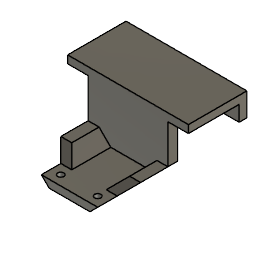
bumper_mount (Autodesk Fusion 360 design; units mm, degrees)
Autodesk Fusion 360 part; units mm, degrees
note: some values were not read from the file. Chosen so that the rebuilt part matches the saved one: which face or edge a step refers to; which pieces of a blend or face edit are solid.
sketch "Sketch1" plane through (0, 0, 0) normal (0, 0, 1) x (1, 0, 0)
  line L0 (-50, 46.2078) -> (-41.5, 46.2078)
  line L1 (-41.5, 46.2078) -> (-41.5, 16.2078)
  line L2 (-41.5, 16.2078) -> (-50, 16.2078)
  line L3 (-50, 16.2078) -> (-50, 46.2078)
  line L4 (-41.5, 16.2078) -> (-0.5, 16.2078)
  line L5 (-0.5, 16.2078) -> (-0.5, 21.2078)
  line L6 (-0.5, 21.2078) -> (-41.5, 21.2078)
  line L7 (-41.5, 21.2078) -> (-41.5, 16.2078)
  line L8 (-0.5, 16.2078) -> (8, 16.2078)
  line L9 (8, 16.2078) -> (8, 46.2078)
  line L10 (8, 46.2078) -> (-0.5, 46.2078)
  line L11 (-0.5, 46.2078) -> (-0.5, 16.2078)
  line L12 (-50, 46.2078) -> (-50, 42.2078)
  line L13 (-50, 42.2078) -> (-41.5, 42.2078)
  line L14 (-0.5, 46.2078) -> (-0.5, 42.2078)
  line L15 (-0.5, 42.2078) -> (8, 42.2078)
  dimension "d1" = 8.5
  dimension "d2" = 30
  dimension "d3" = 41
  dimension "d4" = 5
  dimension "d5" = 8.5
  dimension "d6" = 30
  dimension "d7" = 4
  dimension "d8" = 4
  constraint horizontal L0
  constraint vertical L1
  constraint horizontal L2
  constraint vertical L3
  constraint horizontal L4
  constraint vertical L5
  constraint horizontal L6
  constraint vertical L7
  constraint horizontal L8
  constraint vertical L9
  constraint horizontal L10
  constraint vertical L11
  constraint perpendicular L0 L12
  constraint coincident L1 L13.end
  constraint perpendicular L1 L13
  constraint coincident L11 L14.end
  constraint coincident L9 L15.end
  constraint perpendicular L9 L15
  measures "d1" distance of L0.start L0.end
  measures "d2" distance of L0.start L2.end
  measures "d3" distance of L1.end L4.end
  measures "d4" distance of L1.end L6.end
  measures "d5" distance of L4.end L8.end
  measures "d6" distance of L4.end L10.end
  measures "d7" distance of L0.start L12.end
  measures "d8" distance of L10.end L14.end
extrude "Extrude1" add sketch "Sketch1" against normal blind 8 contours L0 L1 L3 L12 L13 | L9 L10 L11 L14 L15 makes body 1 at (-47.1667, 46.2078, -2.6667) makes body 2 at (5.1667, 46.2078, -2.6667)
extrude "Extrude2" add sketch "Sketch1" along normal blind 4 contours L0 L1 L3 L12 L13 | L1 L2 L3 L7 L13 | L5 L8 L9 L11 L15 | L9 L10 L11 L14 L15 bodies 1 2
extrude "Extrude3" add sketch "Sketch1" along normal blind 4 contours L1 L4 L5 L6 L7 L11 bodies 1 2
sketch "Sketch2" plane through (0, 42.2078, 0) normal (0, -1, 0) x (1, 0, 0)
  line L0 (-41.5, 0) -> (-50, 0)
  line L1 (-50, 0) -> (-50, -8)
  line L2 (-50, -8) -> (-41.5, -8)
  line L3 (-41.5, -8) -> (-41.5, 0)
  line L4 (-50, -8) -> (-50, -7)
  line L5 (-50, 4) -> (-52, 4)
  line L6 (-52, 4) -> (-52, -8)
  line L7 (-52, -8) -> (-50, -8)
  line L8 (8, -8) -> (10, -8)
  line L9 (10, -8) -> (10, 4)
  line L10 (10, 4) -> (8, 4)
  line L11 (8, 4) -> (8, -8)
  line L12 (-50, 4) -> (-50, -8)
  dimension "d15" = 2
  constraint coincident L1.end L2.start
  constraint coincident L1 L4.end
  constraint perpendicular L2 L4
  constraint perpendicular L1 L5
  constraint perpendicular L0 L6
  constraint perpendicular L4 L7
  constraint perpendicular L1 L8
  constraint perpendicular L8 L9
  constraint perpendicular L9 L10
  constraint perpendicular L8 L11
  measures "d15" distance of L5.start L5.end
extrude "Extrude4" add sketch "Sketch2" against normal blind 4 contours L1 L4 L5 L6 L7 L12 | L8 L9 L10 L11 bodies 1
extrude "Extrude5" add sketch "Sketch2" along normal blind 26 contours L1 L4 L5 L6 L7 L12 | L8 L9 L10 L11 bodies 1
chamfer "Chamfer1" distance 8 distance2 26 2 edges at (-51, 16.2078, -8) (9, 16.2078, -8) measured on face at (-30.6667, 16.2078, 2.6667) measured on face at (-30.6667, 16.2078, 2.6667) on bodies 1
sketch "Sketch3" plane through (0, 16.2078, 0) normal (0, -1, 0) x (1, 0, 0)
  line L0 (8, 0) -> (10, 0)
  line L1 (10, 0) -> (10, 4)
  line L2 (10, 4) -> (-52, 4)
  line L3 (-52, 4) -> (-52, 0)
  line L4 (-52, 0) -> (-50, 0)
  line L5 (-50, 0) -> (8, 0)
  line L6 (-52, 4) -> (-26, 4)
  line L7 (-26, 4) -> (-16, 4)
  line L8 (-16, 4) -> (-16, 0)
  line L9 (-16, 0) -> (-26, 0)
  line L10 (-26, 0) -> (-26, 4)
  line L11 (-26, 1) -> (-24, 1)
  line L12 (-24, 1) -> (-24, 3)
  line L13 (-24, 3) -> (-26, 3)
  line L14 (-26, 1) -> (-26, 3)
  line L15 (-16, 1) -> (-18, 1)
  line L16 (-18, 3) -> (-18, 1)
  line L17 (-18, 3) -> (-16, 3)
  line L18 (-16, 3) -> (-16, 1)
  dimension "d22" = 26
  dimension "d23" = 10
  constraint coincident L2.end L3.start
  constraint perpendicular L3 L6
  constraint horizontal L7
  constraint vertical L8
  constraint horizontal L9
  constraint vertical L10
  constraint coincident L10 L11.start
  constraint perpendicular L10 L11
  constraint perpendicular L11 L12
  constraint coincident L10 L13.end
  constraint perpendicular L10 L13
  constraint coincident L8 L15.start
  constraint perpendicular L8 L15
  constraint perpendicular L15 L16
  constraint coincident L8 L17.end
  constraint perpendicular L8 L17
  measures "d22" distance of L2.end L6.end
  measures "d23" distance of L6.end L7.end
extrude "Extrude6" add sketch "Sketch3" along normal blind 1 contours L2 L3 L4 L5 L6 L10 L14 bodies 1
extrude "Extrude7" cut 1 faces at (-43.3333, 15.2078, 2.6667) along direction (0, 1, 0) blind 1 on bodies 1 bodies 1
delete_face "DeleteFace7" 2 faces at (-50, 33.5412, -2.6667) (-51.3333, 33.5412, -5.3333) on bodies 1
delete_face "DeleteFace8" 1 faces at (8, 33.5412, -2.6667) on bodies 1
extrude "Extrude40" add 1 faces at (-14.1667, 21.2078, 1.3333) along direction (0, 1, 0) blind 25 on bodies 1 bodies 1
sketch "Sketch35" plane through (0, 0, 0) normal (0, 0, -1) x (1, 0, 0)
  line L0 (-0.5, -42.2078) -> (10, -42.2078)
  line L1 (10, -42.2078) -> (10, -16.2078)
  line L2 (10, -16.2078) -> (-52, -16.2078)
  line L3 (-52, -16.2078) -> (-52, -42.2078)
  line L4 (-52, -42.2078) -> (-41.5, -42.2078)
  line L5 (-41.5, -42.2078) -> (-41.5, -46.2078)
  line L6 (-41.5, -46.2078) -> (-0.5, -46.2078)
  line L7 (-0.5, -46.2078) -> (-0.5, -42.2078)
  line L8 (-0.5, -16.2078) -> (-41.5, -16.2078)
  line L9 (-41.5, -16.2078) -> (-41.5, -21.2078)
  line L10 (-41.5, -21.2078) -> (-0.5, -21.2078)
  line L11 (-0.5, -21.2078) -> (-0.5, -16.2078)
  dimension "d274" = 5
  constraint horizontal L8
  constraint coincident L2 L8.start
  constraint vertical L4.end L8.end
  constraint vertical L0.start L8.start
  constraint perpendicular L8 L9
  constraint perpendicular L7 L10
  constraint perpendicular L2 L11
  measures "d274" distance of L8.end L9.end
extrude "Extrude41" add sketch "Sketch35" along normal blind 30 contours L2 L8 L9 L10 L11 bodies 1
chamfer "Chamfer2" distance 10 angle 45 2 edges at (-41.5, 18.7078, -30) (-0.5, 18.7078, -30) on bodies 1
sketch "Sketch36" plane through (0, 16.2078, 0) normal (0, -1, 0) x (1, 0, 0)
  line L0 (-10.5, -30) -> (-0.5, -20)
  line L1 (-0.5, -20) -> (-0.5, 0)
  line L2 (-0.5, 0) -> (10, 0)
  line L3 (10, 0) -> (10, 4)
  line L4 (10, 4) -> (-52, 4)
  line L5 (-52, 4) -> (-52, 0)
  line L6 (-52, 0) -> (-41.5, 0)
  line L7 (-41.5, 0) -> (-41.5, -20)
  line L8 (-41.5, -20) -> (-31.5, -30)
  line L9 (-31.5, -30) -> (-10.5, -30)
  line L10 (-41.5, -20) -> (-31.5, -30)
  line L11 (-10.5, -30) -> (-0.5, -20)
  line L12 (-10.5, -30) -> (-31.5, -30)
  line L13 (-41.5, -20) -> (-35.8431, -20)
  line L14 (-35.8431, -20) -> (-29.8431, -26)
  line L15 (-29.8431, -26) -> (-12.1569, -26)
  line L16 (-12.1569, -26) -> (-6.1569, -20)
  line L17 (-6.1569, -20) -> (-0.5, -20)
  dimension "d278" = 4
  dimension "d279" = 4
  constraint coincident L7.end L8.start
  constraint coincident L8.end L9.start
  constraint coincident L0.start L9.end
  constraint coincident L0.end L1.start
  constraint perpendicular L7 L13
  constraint parallel L8 L14
  constraint perpendicular L7 L15
  constraint parallel L15 L17
  constraint parallel L11 L16
  constraint equal L13 L17
  measures "d278" distance of L10 L14
  measures "d279" distance of L12 L15
extrude "Extrude42" add sketch "Sketch36" along normal blind 20 contours L0 L8 L9 L10 L11 L12 L13 L14 L15 L16 L17 bodies 1
chamfer "Chamfer3" distance 6 angle 45 2 edges at (-38.6716, -3.7922, -20) (-3.3284, -3.7922, -20) on bodies 1
extrude "Extrude43" add 1 faces at (-18.0523, -3.7922, -28.6667) along direction (0, -1, 0) blind 10 on bodies 1 bodies 1
sketch "Sketch37" plane through (0, 0, -26) normal (0, 0, 1) x (-1, 0, 0)
  line L0 (12.1569, -16.2078) -> (29.8431, -16.2078)
  line L1 (29.8431, -16.2078) -> (29.8431, 3.7922)
  line L2 (29.8431, 3.7922) -> (35.5, 3.7922)
  line L3 (35.5, 3.7922) -> (35.5, 13.7922)
  line L4 (35.5, 13.7922) -> (6.5, 13.7922)
  line L5 (6.5, 13.7922) -> (6.5, 3.7922)
  line L6 (6.5, 3.7922) -> (12.1569, 3.7922)
  line L7 (12.1569, 3.7922) -> (12.1569, -16.2078)
  point P0 (30.5, 8.7922)
  point P1 (11.5, 8.7922)
  dimension "d285" = 5
  dimension "d286" = 5
  dimension "d287" = 5
  dimension "d288" = 5
  measures "d285" distance of L4 P0
  measures "d286" distance of L3 P0
  measures "d287" distance of L5 P1
  measures "d288" distance of L4 P1
sketch "Sketch38" plane through (0, 46.2078, 0) normal (0, 1, 0) x (-1, 0, 0)
  line L0 (-10, 4) -> (-10, -8)
  line L1 (-10, -8) -> (0.5, -8)
  line L2 (0.5, -8) -> (0.5, 0)
  line L3 (0.5, 0) -> (41.5, 0)
  line L4 (41.5, 0) -> (41.5, -8)
  line L5 (41.5, -8) -> (52, -8)
  line L6 (52, -8) -> (52, 4)
  line L7 (52, 4) -> (-10, 4)
  point P0 (-3.75, -4)
  point P1 (45.75, -4)
  dimension "d289" = 4.25
  dimension "d290" = 4
  dimension "d291" = 4.25
  dimension "d292" = 4
  measures "d289" distance of L2 P0
  measures "d290" distance of L1 P0
  measures "d291" distance of L4 P1
  measures "d292" distance of L5 P1
hole "Hole1" at (3.75, 46.2078, -4) at (-45.75, 46.2078, -4) direction (0, -1, 0) diameter 3.2 end up to surface (4 mm away) bodies 1
hole "Hole2" at (-30.5, -8.7922, -26) at (-11.5, -8.7922, -26) direction (0, 0, -1) diameter 3.2 end up to surface (4 mm away) bodies 1
